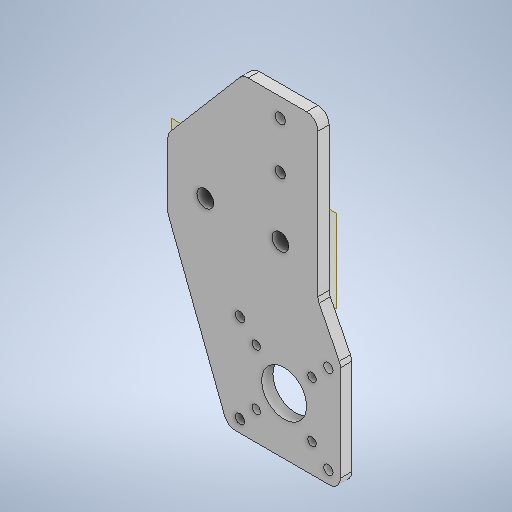
# Autodesk Inventor part: 6MM_ENDPLATE_MOTORMOUNT
Saved by Autodesk Inventor 2025.2 (Build 292293000, 293)
## iProperties
Created: 2026-02-06
Part Number: 6MM_ENDPLATE_MOTORMOUNT
Material: Generic
Document SubType Name: Modeling
Designer: composite
Density: 1 g/cm^3
Appearance: Default
Author: composite
Autodesk Inventor part; units mm, degrees
ref_plane "YZ Plane" through (0, 0, 0) normal (1, 0, 0) x (0, 1, 0)
ref_plane "XZ Plane" through (0, 0, 0) normal (0, 1, 0) x (-1, 0, 0)
ref_plane "XY Plane" through (0, 0, 0) normal (0, 0, 1) x (1, 0, 0)
ref_plane "Work Plane1" through (0, 0, 0) normal (0, 0, 1) x (1, 0, 0)
sketch "Sketch1" plane through (0, 0, 0) normal (0, 0, 1) x (1, 0, 0)
  circle A0 centre (-20, 0.0045) radius 3.4 projected
  circle A1 centre (20, 0.0045) radius 3.4 projected
  line L0 (36.83, 356.5045) -> (36.83, 20.0045) projected
  line L1 (40, 356.5045) -> (40, 20.0045) projected
  line L2 (0, 356.5045) -> (0, 20.0045) projected
  arc A2 (-14.37, -15.6755) -> (-15.94, -17.2455) centre (-14.37, -17.2455) ccw projected
  line L3 (-15.94, -17.2455) -> (-15.94, -18.4255) projected
  arc A3 (-15.94, -18.4255) -> (-14.37, -19.9955) centre (-14.37, -18.4255) ccw projected
  line L4 (-14.37, -19.9955) -> (14.37, -19.9955) projected
  arc A4 (14.37, -19.9955) -> (15.94, -18.4255) centre (14.37, -18.4255) ccw projected
  line L5 (15.94, -18.4255) -> (15.94, -17.2455) projected
  arc A5 (15.94, -17.2455) -> (14.37, -15.6755) centre (14.37, -17.2455) ccw projected
  line L6 (14.37, -15.6755) -> (11.285, -15.6755) projected
  arc A6 (9.715, -14.1055) -> (11.285, -15.6755) centre (11.285, -14.1055) ccw projected
  line L7 (9.715, -14.1055) -> (9.715, -13.6501) projected
  arc A7 (9.9376, -13.1127) -> (9.715, -13.6501) centre (10.475, -13.6501) ccw projected
  line L8 (9.9376, -13.1127) -> (13.6905, -9.3598) projected
  arc A8 (16.6585, -7.6955) -> (13.6905, -9.3598) centre (17.3435, -12.3959) ccw projected
  line L9 (16.6585, -7.6955) -> (23.3415, -7.6955) projected
  arc A9 (26.3095, -9.3598) -> (23.3415, -7.6955) centre (22.6565, -12.3959) ccw projected
  line L10 (26.3095, -9.3598) -> (30.0624, -13.1127) projected
  arc A10 (30.285, -13.6501) -> (30.0624, -13.1127) centre (29.525, -13.6501) ccw projected
  line L11 (30.285, -13.6501) -> (30.285, -14.1055) projected
  arc A11 (28.715, -15.6755) -> (30.285, -14.1055) centre (28.715, -14.1055) ccw projected
  line L12 (28.715, -15.6755) -> (25.63, -15.6755) projected
  arc A12 (25.63, -15.6755) -> (24.06, -17.2455) centre (25.63, -17.2455) ccw projected
  line L13 (24.06, -17.2455) -> (24.06, -18.4345) projected
  arc A13 (24.06, -18.4345) -> (25.797, -19.9955) centre (25.63, -18.4345) ccw projected
  line L14 (25.797, -19.9955) -> (37.0574, -19.9955) projected
  arc A14 (37.0574, -19.9955) -> (40, -16.8255) centre (36.83, -16.8337) ccw projected
  line L15 (40, -16.8255) -> (40, -5.5651) projected
  arc A15 (40, -5.5651) -> (38.43, -4.0555) centre (38.4312, -5.6255) ccw projected
  line L16 (38.43, -4.0555) -> (37.25, -4.0555) projected
  arc A16 (37.25, -4.0555) -> (35.68, -5.6255) centre (37.25, -5.6255) ccw projected
  line L17 (35.68, -5.6255) -> (35.68, -8.7105) projected
  arc A17 (34.111, -10.3353) -> (35.68, -8.7105) centre (34.111, -8.7653) ccw projected
  line L18 (34.111, -10.3353) -> (33.7093, -10.3353) projected
  arc A18 (33.1719, -10.1127) -> (33.7093, -10.3353) centre (33.7093, -9.5753) ccw projected
  line L19 (33.1719, -10.1127) -> (28.9155, -5.8563) projected
  arc A19 (27.7159, -2.4976) -> (28.9155, -5.8563) centre (32.4617, -2.6961) ccw projected
  line L20 (27.7159, -2.4976) -> (27.7159, 2.5754) projected
  arc A20 (29.0111, 5.9609) -> (27.7159, 2.5754) centre (32.4643, 2.6992) ccw projected
  line L21 (29.0111, 5.9609) -> (33.1135, 10.0633) projected
  arc A21 (33.6509, 10.2859) -> (33.1135, 10.0633) centre (33.6509, 9.5259) ccw projected
  line L22 (33.6509, 10.2859) -> (34.11, 10.2859) projected
  arc A22 (35.68, 8.7159) -> (34.11, 10.2859) centre (34.11, 8.7159) ccw projected
  line L23 (35.68, 8.7159) -> (35.68, 5.6309) projected
  arc A23 (35.68, 5.6309) -> (37.1443, 4.0645) centre (37.25, 5.6309) ccw projected
  line L24 (37.1443, 4.0645) -> (38.3243, 4.0645) projected
  arc A24 (38.3243, 4.0645) -> (40, 5.587) centre (38.4306, 5.6308) ccw projected
  line L25 (40, 5.587) -> (40, 16.8451) projected
  arc A25 (40, 16.8451) -> (36.83, 20.0045) centre (36.83, 16.8345) ccw projected
  line L26 (36.83, 20.0045) -> (25.5696, 20.0045) projected
  arc A26 (25.5696, 20.0045) -> (24.06, 18.4356) centre (25.63, 18.4356) ccw projected
  line L27 (24.06, 18.4356) -> (24.06, 17.2545) projected
  arc A27 (24.06, 17.2545) -> (25.63, 15.6845) centre (25.63, 17.2545) ccw projected
  line L28 (25.63, 15.6845) -> (28.715, 15.6845) projected
  arc A28 (30.285, 14.1145) -> (28.715, 15.6845) centre (28.715, 14.1145) ccw projected
  line L29 (30.285, 14.1145) -> (30.285, 13.659) projected
  arc A29 (30.0624, 13.1216) -> (30.285, 13.659) centre (29.525, 13.659) ccw projected
  line L30 (30.0624, 13.1216) -> (25.9081, 8.9673) projected
  arc A30 (22.5494, 7.7045) -> (25.9081, 8.9673) centre (22.6809, 12.4526) ccw projected
  line L31 (22.5494, 7.7045) -> (17.4506, 7.7045) projected
  arc A31 (14.0919, 8.9673) -> (17.4506, 7.7045) centre (17.3191, 12.4526) ccw projected
  line L32 (14.0919, 8.9673) -> (9.9376, 13.1216) projected
  arc A32 (9.715, 13.659) -> (9.9376, 13.1216) centre (10.475, 13.659) ccw projected
  line L33 (9.715, 13.659) -> (9.715, 14.1145) projected
  arc A33 (11.285, 15.6845) -> (9.715, 14.1145) centre (11.285, 14.1145) ccw projected
  line L34 (11.285, 15.6845) -> (14.37, 15.6845) projected
  arc A34 (14.37, 15.6845) -> (15.94, 17.1773) centre (14.3719, 17.2545) ccw projected
  line L35 (15.94, 17.1773) -> (15.94, 18.3573) projected
  arc A35 (15.94, 18.3573) -> (14.3719, 20.0045) centre (14.3719, 18.4345) ccw projected
  line L36 (14.3719, 20.0045) -> (-14.3719, 20.0045) projected
  arc A36 (-14.3719, 20.0045) -> (-15.94, 18.3573) centre (-14.3719, 18.4345) ccw projected
  line L37 (-15.94, 18.3573) -> (-15.94, 17.1773) projected
  arc A37 (-15.94, 17.1773) -> (-14.37, 15.6845) centre (-14.3719, 17.2545) ccw projected
  line L38 (-14.37, 15.6845) -> (-11.285, 15.6845) projected
  arc A38 (-9.715, 14.1145) -> (-11.285, 15.6845) centre (-11.285, 14.1145) ccw projected
  line L39 (-9.715, 14.1145) -> (-9.715, 13.659) projected
  arc A39 (-9.9376, 13.1216) -> (-9.715, 13.659) centre (-10.475, 13.659) ccw projected
  line L40 (-9.9376, 13.1216) -> (-14.0919, 8.9673) projected
  arc A40 (-17.4506, 7.7045) -> (-14.0919, 8.9673) centre (-17.3191, 12.4526) ccw projected
  line L41 (-17.4506, 7.7045) -> (-22.5494, 7.7045) projected
  arc A41 (-25.9081, 8.9673) -> (-22.5494, 7.7045) centre (-22.6809, 12.4526) ccw projected
  line L42 (-25.9081, 8.9673) -> (-30.0624, 13.1216) projected
  arc A42 (-30.285, 13.659) -> (-30.0624, 13.1216) centre (-29.525, 13.659) ccw projected
  line L43 (-30.285, 13.659) -> (-30.285, 14.1145) projected
  arc A43 (-28.715, 15.6845) -> (-30.285, 14.1145) centre (-28.715, 14.1145) ccw projected
  line L44 (-28.715, 15.6845) -> (-25.63, 15.6845) projected
  arc A44 (-25.63, 15.6845) -> (-24.06, 17.2545) centre (-25.63, 17.2545) ccw projected
  line L45 (-24.06, 17.2545) -> (-24.06, 18.4356) projected
  arc A45 (-24.06, 18.4356) -> (-25.5696, 20.0045) centre (-25.63, 18.4356) ccw projected
  line L46 (-25.5696, 20.0045) -> (-36.83, 20.0045) projected
  arc A46 (-36.83, 20.0045) -> (-40, 16.8451) centre (-36.83, 16.8345) ccw projected
  line L47 (-40, 16.8451) -> (-40, 5.587) projected
  arc A47 (-40, 5.587) -> (-38.3243, 4.0645) centre (-38.4306, 5.6308) ccw projected
  line L48 (-38.3243, 4.0645) -> (-37.1443, 4.0645) projected
  arc A48 (-37.1443, 4.0645) -> (-35.68, 5.6309) centre (-37.25, 5.6309) ccw projected
  line L49 (-35.68, 5.6309) -> (-35.68, 8.7159) projected
  arc A49 (-34.11, 10.2859) -> (-35.68, 8.7159) centre (-34.11, 8.7159) ccw projected
  line L50 (-34.11, 10.2859) -> (-33.6509, 10.2859) projected
  arc A50 (-33.1135, 10.0633) -> (-33.6509, 10.2859) centre (-33.6509, 9.5259) ccw projected
  line L51 (-33.1135, 10.0633) -> (-29.0111, 5.9609) projected
  arc A51 (-27.7159, 2.5754) -> (-29.0111, 5.9609) centre (-32.4643, 2.6992) ccw projected
  line L52 (-27.7159, 2.5754) -> (-27.7159, -2.4976) projected
  arc A52 (-28.9155, -5.8563) -> (-27.7159, -2.4976) centre (-32.4617, -2.6961) ccw projected
  line L53 (-28.9155, -5.8563) -> (-33.1719, -10.1127) projected
  arc A53 (-33.7093, -10.3353) -> (-33.1719, -10.1127) centre (-33.7093, -9.5753) ccw projected
  line L54 (-33.7093, -10.3353) -> (-34.111, -10.3353) projected
  arc A54 (-35.68, -8.7105) -> (-34.111, -10.3353) centre (-34.111, -8.7653) ccw projected
  line L55 (-35.68, -8.7105) -> (-35.68, -5.6255) projected
  arc A55 (-35.68, -5.6255) -> (-37.25, -4.0555) centre (-37.25, -5.6255) ccw projected
  line L56 (-37.25, -4.0555) -> (-38.43, -4.0555) projected
  arc A56 (-38.43, -4.0555) -> (-40, -5.5651) centre (-38.4312, -5.6255) ccw projected
  line L57 (-40, -5.5651) -> (-40, -16.8255) projected
  arc A57 (-40, -16.8255) -> (-37.0574, -19.9955) centre (-36.83, -16.8337) ccw projected
  line L58 (-37.0574, -19.9955) -> (-25.797, -19.9955) projected
  arc A58 (-25.797, -19.9955) -> (-24.06, -18.4345) centre (-25.63, -18.4345) ccw projected
  line L59 (-24.06, -18.4345) -> (-24.06, -17.2455) projected
  arc A59 (-24.06, -17.2455) -> (-25.63, -15.6755) centre (-25.63, -17.2455) ccw projected
  line L60 (-25.63, -15.6755) -> (-28.715, -15.6755) projected
  arc A60 (-30.285, -14.1055) -> (-28.715, -15.6755) centre (-28.715, -14.1055) ccw projected
  line L61 (-30.285, -14.1055) -> (-30.285, -13.6501) projected
  arc A61 (-30.0624, -13.1127) -> (-30.285, -13.6501) centre (-29.525, -13.6501) ccw projected
  line L62 (-30.0624, -13.1127) -> (-26.3095, -9.3598) projected
  arc A62 (-23.3415, -7.6955) -> (-26.3095, -9.3598) centre (-22.6565, -12.3959) ccw projected
  line L63 (-23.3415, -7.6955) -> (-16.6585, -7.6955) projected
  arc A63 (-13.6905, -9.3598) -> (-16.6585, -7.6955) centre (-17.3435, -12.3959) ccw projected
  line L64 (-13.6905, -9.3598) -> (-9.9376, -13.1127) projected
  arc A64 (-9.715, -13.6501) -> (-9.9376, -13.1127) centre (-10.475, -13.6501) ccw projected
  line L65 (-9.715, -13.6501) -> (-9.715, -14.1055) projected
  arc A65 (-11.285, -15.6755) -> (-9.715, -14.1055) centre (-11.285, -14.1055) ccw projected
  line L66 (-11.285, -15.6755) -> (-14.37, -15.6755) projected
  circle A66 centre (20, 0.0045) radius 3.4 projected
  circle A67 centre (-20, 0.0045) radius 3.4 projected
  arc A68 (-5.7137, 11.236) -> (-5.3418, 12.1341) centre (-6.6118, 12.1341) ccw projected
  line L67 (-5.3418, 12.1341) -> (-5.3418, 14.4145) projected
  arc A69 (-4.0718, 15.6845) -> (-5.3418, 14.4145) centre (-4.0718, 14.4145) ccw projected
  line L68 (-4.0718, 15.6845) -> (4.0718, 15.6845) projected
  arc A70 (5.3418, 14.4145) -> (4.0718, 15.6845) centre (4.0718, 14.4145) ccw projected
  line L69 (5.3418, 14.4145) -> (5.3418, 12.1341) projected
  arc A71 (5.3418, 12.1341) -> (5.7137, 11.236) centre (6.6118, 12.1341) ccw projected
  line L70 (5.7137, 11.236) -> (10.5988, 6.351) projected
  arc A72 (12.2841, 3.2635) -> (10.5988, 6.351) centre (7.5685, 2.6931) ccw projected
  line L71 (12.2841, 3.2635) -> (12.2841, -2.7205) projected
  arc A73 (11.2012, -5.7396) -> (12.2841, -2.7205) centre (7.5341, -2.7205) ccw projected
  line L72 (11.2012, -5.7396) -> (5.7137, -11.2271) projected
  arc A74 (5.7137, -11.2271) -> (5.3418, -12.1251) centre (6.6118, -12.1251) ccw projected
  line L73 (5.3418, -12.1251) -> (5.3418, -14.4055) projected
  arc A75 (4.0718, -15.6755) -> (5.3418, -14.4055) centre (4.0718, -14.4055) ccw projected
  line L74 (4.0718, -15.6755) -> (-4.0718, -15.6755) projected
  arc A76 (-5.3418, -14.4055) -> (-4.0718, -15.6755) centre (-4.0718, -14.4055) ccw projected
  line L75 (-5.3418, -14.4055) -> (-5.3418, -12.1251) projected
  arc A77 (-5.3418, -12.1251) -> (-5.7137, -11.2271) centre (-6.6118, -12.1251) ccw projected
  line L76 (-5.7137, -11.2271) -> (-11.2012, -5.7396) projected
  arc A78 (-12.2841, -2.7205) -> (-11.2012, -5.7396) centre (-7.5341, -2.7205) ccw projected
  line L77 (-12.2841, -2.7205) -> (-12.2841, 3.2635) projected
  arc A79 (-10.5988, 6.351) -> (-12.2841, 3.2635) centre (-7.5685, 2.6931) ccw projected
  line L78 (-10.5988, 6.351) -> (-5.7137, 11.236) projected
  line L79 (0, -53.9955) -> (0, -47.9955) projected
  line L80 (-8, -53.9955) -> (-35.1674, -53.9955) projected
  line L81 (47, -83.9955) -> (47, -53.9955)
  line L82 (-3, -83.9955) -> (47, -83.9955)
  point P0 (0, 0)
  point P1 (22, -68.9955)
  constraints: 4 end point, 1 horizontal, 1 vertical, 4 other
sketch "Sketch2" plane through (0, 0, 0) normal (0, 0, 1) x (1, 0, 0)
  circle A0 centre (20, 32.0045) radius 2.75
  circle A1 centre (20, 57.0045) radius 2.75
  line L0 (40, 5.587) -> (40, 16.8451) projected
  line L1 (40, -16.8255) -> (40, -5.5651) projected
  line L2 (25.797, -19.9955) -> (37.0574, -19.9955) projected
  line L3 (-14.37, -19.9955) -> (14.37, -19.9955) projected
  line L4 (-40, -5.5651) -> (-40, -16.8255) projected
  line L5 (-8, -53.9955) -> (-35.1674, -53.9955) projected
  line L6 (0, -53.9955) -> (0, -47.9955) construction
  line L7 (40, 356.5045) -> (40, 20.0045) projected
  line L8 (47, -83.9955) -> (47, -53.9955) construction
  line L9 (-3, -83.9955) -> (47, -83.9955) construction
  line L10 (47, -83.9955) -> (47, -53.9955) construction
  line L11 (-3, -83.9955) -> (47, -83.9955) construction
  line L12 (0, 356.5045) -> (0, 20.0045) projected
  line L13 (-40, 20.0045) -> (0, 67.0045)
  line L14 (0, 67.0045) -> (40, 67.0045)
  line L15 (47, -53.9955) -> (52, -53.9955) construction
  line L16 (43, -89.9955) -> (43, -47.9955) construction
  line L17 (1, -47.9955) -> (1, -89.9955) construction
  circle A2 centre (-20, 0.0045) radius 4.5
  circle A3 centre (20, 0.0045) radius 4.5
  line L18 (-25.5696, 20.0045) -> (-36.83, 20.0045) projected
  line L19 (-36.83, 20.0045) -> (-40, 20.0045) construction
  line L20 (-6.2, -40.7955) -> (50.2, -40.7955) construction
  line L21 (50.2, -40.7955) -> (50.2, -97.1955) construction
  line L22 (50.2, -97.1955) -> (-6.2, -97.1955) construction
  line L23 (-6.2, -97.1955) -> (-6.2, -40.7955) construction
  line L24 (-6.2, -40.7955) -> (50.2, -97.1955) construction
  line L25 (50.2, -40.7955) -> (-6.2, -97.1955) construction
  line L26 (40, 67.0045) -> (40, -16.8255)
  line L27 (52, -53.9955) -> (52, -40.7955)
  line L28 (52, -40.7955) -> (40, -16.8255)
  line L29 (52, -99.1955) -> (-8.2, -99.1955)
  line L30 (-8.2, -99.1955) -> (-40, -16.8255)
  line L31 (-40, -16.8255) -> (-40, 20.0045)
  line L32 (52, -99.1955) -> (52, -53.9955)
  point P0 (0, 0)
  point P1 (40, 11.216)
  point P2 (22, -68.9955)
  point P3 (40, 20.0045)
  dimension "d0" = 5.5
  dimension "d1" = 20
  dimension "d2" = 12
  dimension "d3" = 25
  dimension "d7" = 5
  dimension "d10" = 9
  dimension "d11" = 9
  dimension "d34" = 56.4
  dimension "d35" = 56.4
  dimension "d36" = 2
  dimension "d37" = 2
  dimension "d38" = 10
  constraints: 46 end point, 6 vertical, 4 centre point, 3 horizontal, 3 midpoint, 3 parallel, 2 coincident, 2 collinear, 2 horizontal alignment, 2 perpendicular, 2 point on line, 1 equal radius, 1 vertical alignment, 8 other
  measures "d0" diameter of A0
  measures "d1" horizontal distance of point (40, 11.216) A1.centre
  measures "d2" vertical distance of A0.centre L7.end
  measures "d3" distance of A0.centre A1.centre
  measures "d7" distance of L8.end L15.end
  measures "d10" diameter of A2
  measures "d11" diameter of A3
  measures "d34" distance of L20.end L21.end
  measures "d35" distance of L21.end L22.end
  measures "d36" distance between parallel lines of L29 L22
  measures "d37" distance from line of L29.end L23
  measures "d38" distance from line of L14 A1.centre
extrude "Extrusion1" add sketch "Sketch2" along normal blind 6
fillet "Fillet1" radius 6 8 edges at (-40, -16.8255, 3) (-40, 20.0045, 3) (0, 67.0045, 3) (52, -40.7955, 3) (52, -99.1955, 3) (-8.2, -99.1955, 3) (40, -16.8255, 3) (40, 67.0045, 3)
sketch "Sketch3" plane through (0, 0, 0) normal (0, 0, -1) x (-1, 0, 0)
  circle A0 centre (-22, -68.9955) radius 21 construction
  circle A1 centre (-7.1508, -54.1463) radius 2.25
  circle A2 centre (-36.8492, -54.1463) radius 2.25
  circle A3 centre (-36.8492, -83.8448) radius 2.25
  circle A4 centre (-7.1508, -83.8448) radius 2.25
  circle A5 centre (-22, -68.9955) radius 33.333
  circle A6 centre (1.57, -92.5655) radius 2.5
  circle A7 centre (1.57, -45.4255) radius 2.5
  circle A8 centre (-45.57, -45.4255) radius 2.5
  circle A9 centre (-45.57, -92.5655) radius 2.5
  circle A10 centre (-22, -68.9955) radius 12
  point P0 (0, 0)
  dimension "d22" = 42
  dimension "d25" = 360
  dimension "d27" = 4.5
  dimension "d30" = 360
  dimension "d32" = 47.14
  dimension "d33" = 5
  dimension "d40" = 24
  constraints: 9 centre point, 3 coincident, 1 horizontal alignment, 1 vertical alignment, 24 other
  measures "d27" diameter of A1
  measures "d32" distance of A6.centre A7.centre
  measures "d33" diameter of A6
  measures "d40" diameter of A10
extrude "Extrusion2" cut sketch "Sketch3" against normal blind 6 contours A1 | A2 | A3 | A4 | A7 A5 | A5 A7 | A6 A5 | A5 A6 | A8 A5 | A5 A8 | A9 A5 | A5 A9 | A10
equation "\"d11\" = d10"
body "Solid1"
